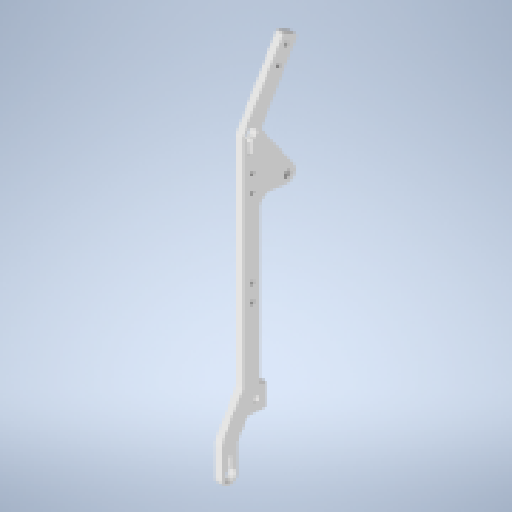
# Autodesk Inventor part: Door Lower Parallel Bar
Saved by Autodesk Inventor 2024 (Build 280153000, 153)
## iProperties
Created: 2024-08-28
Part Number: Door Lower Parallel Bar
Material: Generic
Document SubType Name: Modeling
Designer: Ishaan
Density: 1 g/cm^3
Appearance: Default
Mass: 27.6729 g
Surface Area: 140.766 cm^2
Volume: 27.6729 cm^3
Author: Ishaan
Autodesk Inventor part; units mm, degrees
ref_plane "YZ Plane" through (0, 0, 0) normal (1, 0, 0) x (0, 1, 0)
ref_plane "XZ Plane" through (0, 0, 0) normal (0, 1, 0) x (-1, 0, 0)
ref_plane "XY Plane" through (0, 0, 0) normal (0, 0, 1) x (1, 0, 0)
sketch "Sketch1" plane through (0, 0, 0) normal (1, 0, 0) x (0, 1, 0)
  line L0 (-10, -10) -> (10, -10) construction
  line L1 (10, -10) -> (10, 10) construction
  line L2 (10, 10) -> (-10, 10) construction
  line L3 (-10, 10) -> (-10, -10) construction
  line L4 (-10, -10) -> (10, 10) construction
  line L5 (10, -10) -> (-10, 10) construction
  line L6 (270, -20) -> (66.6603, -20)
  circle A0 centre (24.2487, -14) radius 5 construction
  line L7 (0, 0) -> (24.2487, -14) construction
  line L8 (0, 0) -> (24.2487, 0)
  line L9 (31.2487, -1.8756) -> (59.1603, -17.9904)
  arc A1 (31.2487, -1.8756) -> (24.2487, 0) centre (24.2487, -14) ccw
  arc A2 (59.1603, -17.9904) -> (66.6603, -20) centre (66.6603, -5) ccw
  dimension "d0" = 270
  dimension "d1" = 20
  dimension "d4" = 20
  dimension "d5" = 20
  dimension "d112" = 10
  dimension "d113" = 28
  dimension "d114" = 150
  dimension "d116" = 15
  dimension "d118" = 9
  constraints: 21 end point, 4 point on circle, 4 tangent, 3 centre point, 3 horizontal, 3 parallel, 2 midpoint, 1 coincident, 1 concentric, 1 perpendicular
  measures "d0" horizontal distance of point (0, 0) L6.start
  measures "d1" vertical distance of L7.start L6.start
  measures "d4" distance of L2.end L1.end
  measures "d5" distance of L1.end L0.end
  measures "d112" diameter of A0
  measures "d113" distance of L7.end point (0, 0)
  measures "d114" angle of L6 L7
  measures "d116" radius of A2
  measures "d118" distance edge to line of A0 L9
surface extrude "ExtrusionSrf1" sketch "Sketch1" along normal mid plane 6.35 shown no curves L6 A2 L9 A1 L8
thicken "Thicken1" operation new thickness 16 both sides yes extend neighbours no toward (0, 0, -1) faces at (-1.0583, 202.2201, -20) (1.0583, 62.3582, -19.3698) (1.0583, 49.8564, -12.6188) (-1.0583, 30.5319, -1.4891) (-1.0583, 16.1658, 0)
sketch "Sketch2" plane through (3.175, 39.0333, -31) normal (1, 0, 0) x (0, 0, -1)
  line L0 (4, 0.9667) -> (-16, 0.9667)
  line L1 (-16, 0.9667) -> (-16, 20.9667)
  line L2 (-16, 20.9667) -> (4, 20.9667)
  line L3 (4, 20.9667) -> (4, 0.9667)
  line L4 (4, 0.9667) -> (-16, 20.9667) construction
  line L5 (-16, 0.9667) -> (4, 20.9667) construction
  line L6 (-39, -39.0333) -> (-23, -39.0333) projected
  line L7 (-39, -39.0333) -> (-23, -39.0333) projected
  circle A0 centre (-31, -39.0333) radius 8
  line L8 (-19, 230.9667) -> (-3, 230.9667) projected
  circle A1 centre (-11, 230.9667) radius 8
  line L9 (-19, 27.6269) -> (-19, 230.9667) projected
  point P0 (-6, 10.9667)
  point P1 (-6, 10.9667)
  dimension "d75" = 20
  dimension "d76" = 20
  dimension "d78" = 50
  dimension "d119" = 3
  constraints: 12 end point, 4 midpoint, 3 coincident, 2 parallel, 1 horizontal, 1 perpendicular, 6 other
  measures "d75" distance of L1.end L2.end
  measures "d76" distance of L0.end L1.end
  measures "d78" vertical distance of point (-6, 10.967) point (-31, -39.033)
  measures "d119" distance between parallel lines of L1 L9
extrude "Extrusion1" add sketch "Sketch2" against normal up to surface (6.35 mm away) contours L0 L1 L2 L3 | L6 A0 | A1 L8 picked at (-30.6786, -41.6805) picked at (-8.4108, 231.6049)
fillet "Fillet1" radius 1 2 edges at (0, 60, -35) (0, 40, -35)
hole "Hole2" at (3.175, 50, -25) direction (-1, 0, 0) diameter 5.3 end through all
hole "Hole3" at (3.175, 0, 0) at (3.175, 270, -20) direction (-1, 0, 0) diameter 11.05 end through all
sketch "Sketch4" plane through (3.175, 270, -20) normal (1, 0, 0) x (0, 0, -1)
  line L0 (-20, -270) -> (-20, -255) construction
  line L1 (-18.5, -270) -> (-18.5, -255)
  line L2 (-21.5, -255) -> (-21.5, -270)
  arc A0 (-21.5, -270) -> (-18.5, -270) centre (-20, -270) ccw
  arc A1 (-18.5, -255) -> (-21.5, -255) centre (-20, -255) ccw
  line L3 (0, 0) -> (0, -15) construction
  line L4 (1.5, 0) -> (1.5, -15)
  line L5 (-1.5, -15) -> (-1.5, 0)
  arc A2 (1.5, 0) -> (-1.5, 0) centre (0, 0) ccw
  arc A3 (-1.5, -15) -> (1.5, -15) centre (0, -15) ccw
  point P0 (-20, -262.5)
  point P1 (0, -7.5)
  dimension "d63" = 15
  dimension "d64" = 3
  constraints: 16 end point, 8 point on circle, 8 tangent, 4 centre point, 3 parallel, 2 midpoint, 2 vertical, 1 coincident, 1 equal radius
  measures "d63" distance of L0.start L0.end
  measures "d64" diameter of A1
extrude "Extrusion2" cut sketch "Sketch4" against normal through all
fillet "Fillet2" radius 1 4 edges at (0, 5.3175, 1.5) (0, 5.3175, -1.5) (0, 264.6825, -18.5) (0, 264.6825, -21.5)
sketch "Sketch5" plane through (3.175, 270, -20) normal (1, 0, 0) x (0, 0, -1)
  line L0 (8, -196.2751) -> (8, -5.6951)
  circle A0 centre (5, -220) radius 2.65 projected
  line L1 (8, -203.3397) -> (8, 0) construction
  line L2 (1, -32) -> (1, -48) construction
  line L3 (-8, -203.3397) -> (-8, 0) projected
  line L4 (1, -122) -> (1, -138) construction
  point P0 (1, -40)
  point P1 (1, -40)
  point P2 (1, -130)
  dimension "d132" = 180
  dimension "d133" = 16
  dimension "d134" = 9
  dimension "d135" = 90
  constraints: 6 end point, 3 collinear, 2 midpoint, 2 vertical, 1 coincident
  measures "d132" vertical distance of point (1, -40) A0.centre
  measures "d133" distance of L2.start L2.end
  measures "d134" distance between parallel lines of L3 L2
  measures "d135" distance of point (1, -40) point (1, -130)
hole "Hole4" at (3.175, 132, -21) at (3.175, 148, -21) at (3.175, 222, -21) at (3.175, 238, -21) direction (-1, 0, 0) diameter 4.134 end through all thread size "M5x0.8" class "6H" standard "ANSI Metric M Profile"
fillet "Fillet5" radius 3 2 edges at (0, 60, -27.0146) (0, 40, -16.1658)
sketch "Sketch6" plane through (3.175, 270, -20) normal (1, 0, 0) x (0, 0, -1)
  line L0 (6.5532, 4.5886) -> (52.0457, -60.3814)
  line L1 (52.0457, -60.3814) -> (8, -52.6149)
  circle A0 centre (34.4146, -49.1491) radius 8
  circle A1 centre (1, -32) radius 2.067 projected
  circle A2 centre (1, -48) radius 2.067 projected
  circle A3 centre (1, -122) radius 2.067 projected
  circle A4 centre (1, -138) radius 2.067 projected
  arc A5 (2.1169, -5.1034) -> (1.5, -6.0271) centre (2.5, -6.0271) ccw projected
  line L2 (1.5, -6.0271) -> (1.5, -15) projected
  arc A6 (-1.5, -15) -> (1.5, -15) centre (0, -15) ccw projected
  line L3 (-1.5, -15) -> (-1.5, -6.0271) projected
  arc A7 (-1.5, -6.0271) -> (-2.1169, -5.1034) centre (-2.5, -6.0271) ccw projected
  arc A8 (2.1169, -5.1034) -> (-2.1169, -5.1034) centre (0, 0) ccw projected
  arc A9 (-18.5, -263.9729) -> (-17.8831, -264.8966) centre (-17.5, -263.9729) ccw projected
  arc A10 (-22.1169, -264.8966) -> (-17.8831, -264.8966) centre (-20, -270) ccw projected
  arc A11 (-22.1169, -264.8966) -> (-21.5, -263.9729) centre (-22.5, -263.9729) ccw projected
  line L4 (-21.5, -263.9729) -> (-21.5, -255) projected
  arc A12 (-18.5, -255) -> (-21.5, -255) centre (-20, -255) ccw projected
  line L5 (-18.5, -255) -> (-18.5, -263.9729) projected
  arc A13 (14, -230) -> (15, -229) centre (14, -229) ccw projected
  line L6 (15, -229) -> (15, -211) projected
  arc A14 (15, -211) -> (14, -210) centre (14, -211) ccw projected
  line L7 (14, -210) -> (10.7411, -210) projected
  arc A15 (7.7709, -206.5777) -> (10.7411, -210) centre (10.7411, -207) ccw projected
  arc A16 (7.7709, -206.5777) -> (8, -203.3397) centre (-15, -203.3397) ccw projected
  line L8 (8, -203.3397) -> (8, 0) projected
  arc A17 (8, 0) -> (-8, 0) centre (0, 0) ccw projected
  line L9 (-8, -203.3397) -> (-8, 0) projected
  arc A18 (-8.9378, -206.8397) -> (-8, -203.3397) centre (-15, -203.3397) ccw projected
  line L10 (-25.0526, -234.7513) -> (-8.9378, -206.8397) projected
  arc A19 (-25.0526, -234.7513) -> (-28, -245.7513) centre (-6, -245.7513) ccw projected
  line L11 (-28, -270) -> (-28, -245.7513) projected
  arc A20 (-28, -270) -> (-12, -270) centre (-20, -270) ccw projected
  line L12 (-12, -270) -> (-12, -245.7513) projected
  arc A21 (-11.1962, -242.7513) -> (-12, -245.7513) centre (-6, -245.7513) ccw projected
  line L13 (-11.1962, -242.7513) -> (-4.7002, -231.5) projected
  arc A22 (-2.1021, -230) -> (-4.7002, -231.5) centre (-2.1021, -233) ccw projected
  line L14 (-2.1021, -230) -> (14, -230) projected
  circle A23 centre (5, -220) radius 2.65 projected
  arc A24 (8, 0) -> (-8, 0) centre (0, 0) ccw projected
  point P0 (40.9678, -44.5605)
  point P1 (33.0254, -57.0276)
  point P2 (6.5532, 4.5886)
  point P3 (8, -52.6149)
  dimension "d98" = 16
  dimension "d122" = 80
  dimension "d123" = 60
  dimension "d124" = 35
  constraints: 4 end point, 3 tangent, 1 centre point
  measures "d98" diameter of A0
  measures "d122" angle of L8 L1
  measures "d123" distance of A8.centre A0.centre
  measures "d124" angle of L0 L8
extrude "Extrusion3" add sketch "Sketch6" against normal up to surface (6.35 mm away) contours L0 A0 L1 L8 A17 | A0
fillet "Fillet4" radius 10 1 edges at (0, 217.3851, -28)
sketch "Sketch8" plane through (3.175, 0, 0) normal (1, 0, 0) x (0, 0, -1)
  arc A0 (53.0254, 212.9724) -> (60.9678, 225.4395) centre (54.4146, 220.8509) ccw projected
  point P0 (0, 0)
  constraints: 1 coincident
hole "Hole6" at (3.175, 220.8509, -54.4146) direction (-1, 0, 0) diameter 6.4008 end through all thread size "5/16-18 UNC" class "2B" standard "ANSI Unified Screw Threads"
sketch "Sketch9" plane through (3.175, 0, 0) normal (1, 0, 0) x (0, 0, -1)
  circle A0 centre (54.4146, 220.8509) radius 3.2004 projected
  circle A1 centre (21, 238) radius 2.067 projected
  circle A2 centre (21, 222) radius 2.067 projected
  circle A3 centre (21, 148) radius 2.067 projected
  circle A4 centre (21, 132) radius 2.067 projected
  arc A5 (22.1169, 264.8966) -> (21.5, 263.9729) centre (22.5, 263.9729) ccw projected
  line L0 (21.5, 263.9729) -> (21.5, 255) projected
  arc A6 (18.5, 255) -> (21.5, 255) centre (20, 255) ccw projected
  line L1 (18.5, 255) -> (18.5, 263.9729) projected
  arc A7 (18.5, 263.9729) -> (17.8831, 264.8966) centre (17.5, 263.9729) ccw projected
  arc A8 (22.1169, 264.8966) -> (17.8831, 264.8966) centre (20, 270) ccw projected
  arc A9 (1.5, 6.0271) -> (2.1169, 5.1034) centre (2.5, 6.0271) ccw projected
  arc A10 (-2.1169, 5.1034) -> (2.1169, 5.1034) centre (0, 0) ccw projected
  arc A11 (-2.1169, 5.1034) -> (-1.5, 6.0271) centre (-2.5, 6.0271) ccw projected
  line L2 (-1.5, 6.0271) -> (-1.5, 15) projected
  arc A12 (1.5, 15) -> (-1.5, 15) centre (0, 15) ccw projected
  line L3 (1.5, 15) -> (1.5, 6.0271) projected
  arc A13 (34, 40) -> (35, 41) centre (34, 41) ccw projected
  line L4 (35, 41) -> (35, 59) projected
  arc A14 (35, 59) -> (34, 60) centre (34, 59) ccw projected
  line L5 (34, 60) -> (30.7411, 60) projected
  arc A15 (27.7709, 63.4223) -> (30.7411, 60) centre (30.7411, 63) ccw projected
  arc A16 (27.7709, 63.4223) -> (28, 66.6603) centre (5, 66.6603) ccw projected
  line L6 (28, 66.6603) -> (28, 205.4675) projected
  arc A17 (39.7365, 215.3156) -> (28, 205.4675) centre (38, 205.4675) ccw projected
  line L7 (39.7365, 215.3156) -> (53.0254, 212.9724) projected
  arc A18 (53.0254, 212.9724) -> (60.9678, 225.4395) centre (54.4146, 220.8509) ccw projected
  line L8 (60.9678, 225.4395) -> (26.5532, 274.5886) projected
  arc A19 (26.5532, 274.5886) -> (12, 270) centre (20, 270) ccw projected
  line L9 (12, 66.6603) -> (12, 270) projected
  arc A20 (11.0622, 63.1603) -> (12, 66.6603) centre (5, 66.6603) ccw projected
  line L10 (-5.0526, 35.2487) -> (11.0622, 63.1603) projected
  arc A21 (-5.0526, 35.2487) -> (-8, 24.2487) centre (14, 24.2487) ccw projected
  line L11 (-8, 0) -> (-8, 24.2487) projected
  arc A22 (-8, 0) -> (8, 0) centre (0, 0) ccw projected
  line L12 (8, 0) -> (8, 24.2487) projected
  arc A23 (8.8038, 27.2487) -> (8, 24.2487) centre (14, 24.2487) ccw projected
  line L13 (8.8038, 27.2487) -> (15.2998, 38.5) projected
  arc A24 (17.8979, 40) -> (15.2998, 38.5) centre (17.8979, 37) ccw projected
  line L14 (17.8979, 40) -> (34, 40) projected
  circle A25 centre (25, 50) radius 2.65 projected
  line L15 (66.9282, 335.282) -> (26.9282, 266)
  line L16 (26.9282, 266) -> (13.0718, 274)
  line L17 (13.0718, 274) -> (53.0718, 343.282)
  line L18 (53.0718, 343.282) -> (66.9282, 335.282)
  line L19 (66.9282, 335.282) -> (13.0718, 274) construction
  line L20 (26.9282, 266) -> (53.0718, 343.282) construction
  line L21 (20, 270) -> (60, 339.282) construction
  line L22 (20, 270) -> (60, 339.282) construction
  line L23 (28.6603, 265) -> (68.6603, 334.282) construction
  line L24 (51.3397, 344.282) -> (11.3397, 275) construction
  arc A26 (11.3397, 275) -> (28.6603, 265) centre (20, 270) ccw construction
  arc A27 (68.6603, 334.282) -> (51.3397, 344.282) centre (60, 339.282) ccw construction
  line L25 (11.3399, 284.2002) -> (46.7375, 345.5106) construction
  point P0 (40, 304.641)
  point P1 (40, 304.641)
  point P2 (29.4765, 270.4138)
  point P3 (40, 304.641)
  dimension "d149" = 150
  dimension "d150" = 80
  dimension "d152" = 20
  dimension "d153" = 4.6
  constraints: 24 end point, 7 midpoint, 5 tangent, 4 parallel, 4 point on circle, 2 centre point, 2 perpendicular
  measures "d149" angle of L17 L9
  measures "d150" distance of L21.start L21.end
  measures "d152" diameter of A27
  measures "d153" distance between parallel lines of L24 L25
extrude "Extrusion4" add sketch "Sketch9" against normal up to surface (6.35 mm away) contours L17 L18 L15 L8 A19
fillet "Fillet6" radius 2 1 edges at (0, 270.4138, -29.4765)
fillet "Fillet7" radius 2 2 edges at (0, 343.282, -53.0718) (0, 335.282, -66.9282)
sketch "Sketch10" plane through (3.175, 0, 0) normal (1, 0, 0) x (0, 0, -1)
  circle A0 centre (54.4146, 220.8509) radius 3.2004 projected
  circle A1 centre (21, 238) radius 2.067 projected
  circle A2 centre (21, 222) radius 2.067 projected
  circle A3 centre (21, 148) radius 2.067 projected
  circle A4 centre (21, 132) radius 2.067 projected
  arc A5 (22.1169, 264.8966) -> (21.5, 263.9729) centre (22.5, 263.9729) ccw projected
  line L0 (21.5, 263.9729) -> (21.5, 255) projected
  arc A6 (18.5, 255) -> (21.5, 255) centre (20, 255) ccw projected
  line L1 (18.5, 255) -> (18.5, 263.9729) projected
  arc A7 (18.5, 263.9729) -> (17.8831, 264.8966) centre (17.5, 263.9729) ccw projected
  arc A8 (22.1169, 264.8966) -> (17.8831, 264.8966) centre (20, 270) ccw projected
  arc A9 (1.5, 6.0271) -> (2.1169, 5.1034) centre (2.5, 6.0271) ccw projected
  arc A10 (-2.1169, 5.1034) -> (2.1169, 5.1034) centre (0, 0) ccw projected
  arc A11 (-2.1169, 5.1034) -> (-1.5, 6.0271) centre (-2.5, 6.0271) ccw projected
  line L2 (-1.5, 6.0271) -> (-1.5, 15) projected
  arc A12 (1.5, 15) -> (-1.5, 15) centre (0, 15) ccw projected
  line L3 (1.5, 15) -> (1.5, 6.0271) projected
  arc A13 (65.9282, 333.55) -> (65.1962, 336.282) centre (64.1962, 334.55) ccw projected
  line L4 (65.1962, 336.282) -> (54.8038, 342.282) projected
  arc A14 (54.8038, 342.282) -> (52.0718, 341.55) centre (53.8038, 340.55) ccw projected
  line L5 (52.0718, 341.55) -> (13.0718, 274) projected
  arc A15 (13.0718, 274) -> (12, 270) centre (20, 270) ccw projected
  line L6 (12, 66.6603) -> (12, 270) projected
  arc A16 (11.0622, 63.1603) -> (12, 66.6603) centre (5, 66.6603) ccw projected
  line L7 (-5.0526, 35.2487) -> (11.0622, 63.1603) projected
  arc A17 (-5.0526, 35.2487) -> (-8, 24.2487) centre (14, 24.2487) ccw projected
  line L8 (-8, 0) -> (-8, 24.2487) projected
  arc A18 (-8, 0) -> (8, 0) centre (0, 0) ccw projected
  line L9 (8, 0) -> (8, 24.2487) projected
  arc A19 (8.8038, 27.2487) -> (8, 24.2487) centre (14, 24.2487) ccw projected
  line L10 (8.8038, 27.2487) -> (15.2998, 38.5) projected
  arc A20 (17.8979, 40) -> (15.2998, 38.5) centre (17.8979, 37) ccw projected
  line L11 (17.8979, 40) -> (34, 40) projected
  arc A21 (34, 40) -> (35, 41) centre (34, 41) ccw projected
  line L12 (35, 41) -> (35, 59) projected
  arc A22 (35, 59) -> (34, 60) centre (34, 59) ccw projected
  line L13 (34, 60) -> (30.7411, 60) projected
  arc A23 (27.7709, 63.4223) -> (30.7411, 60) centre (30.7411, 63) ccw projected
  arc A24 (27.7709, 63.4223) -> (28, 66.6603) centre (5, 66.6603) ccw projected
  line L14 (28, 66.6603) -> (28, 205.4675) projected
  arc A25 (39.7365, 215.3156) -> (28, 205.4675) centre (38, 205.4675) ccw projected
  line L15 (39.7365, 215.3156) -> (53.0254, 212.9724) projected
  arc A26 (53.0254, 212.9724) -> (60.9678, 225.4395) centre (54.4146, 220.8509) ccw projected
  line L16 (60.9678, 225.4395) -> (30.2073, 269.37) projected
  arc A27 (30.1136, 271.5172) -> (30.2073, 269.37) centre (31.8456, 270.5172) ccw projected
  line L17 (30.1136, 271.5172) -> (65.9282, 333.55) projected
  circle A28 centre (25, 50) radius 2.65 projected
  line L18 (47, 316.7654) -> (56, 332.3538) construction
  point P0 (60, 339.282)
  dimension "d154" = 18
  dimension "d155" = 8
  dimension "d156" = 8
  constraints: 2 coincident, 2 end point, 1 midpoint, 1 parallel, 1 point on line
  measures "d154" distance of L18.start L18.end
  measures "d155" distance between parallel lines of L18 L5
  measures "d156" distance from line of L4 L18.end
hole "Hole7" at (3.175, 316.7654, -47) at (3.175, 332.3538, -56) direction (-1, 0, 0) diameter 4.134 depth 6.35 thread size "M5x0.8" class "6H" standard "ANSI Metric M Profile"
body "Solid1"
body "Srf1"
